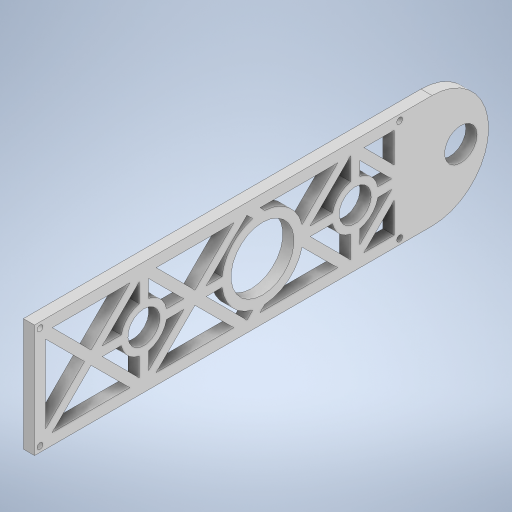
# Autodesk Inventor part: Side_Piece
Saved by Autodesk Inventor 2023 (Build 270158030, 158C)
## iProperties
Created: 2022-06-17
Part Number: Side_Piece
Material: Generic
Document SubType Name: Modeling
Designer: Mlees
Density: 1 g/cm^3
Appearance: Default
Author: Mlees
Autodesk Inventor part; units mm, degrees
ref_plane "YZ Plane" through (0, 0, 0) normal (1, 0, 0) x (0, 1, 0)
ref_plane "XZ Plane" through (0, 0, 0) normal (0, 1, 0) x (-1, 0, 0)
ref_plane "XY Plane" through (0, 0, 0) normal (0, 0, 1) x (1, 0, 0)
sketch "Sketch1" plane through (0, 0, 0) normal (1, 0, 0) x (0, 1, 0)
  line L0 (0, 0) -> (61, 0)
  line L1 (61, 0) -> (61, -200)
  line L2 (61, -200) -> (0, -200)
  line L3 (0, -200) -> (0, 0)
  line L4 (51.4645, -6) -> (9.5355, -6)
  circle A0 centre (30.5, -173) radius 8.625
  circle A1 centre (30.5, -123) radius 17
  circle A2 centre (30.5, -59) radius 8.625
  line L5 (55, -51.4645) -> (55, -9.5355)
  line L6 (55, -9.5355) -> (34.0355, -30.5)
  line L7 (6, -9.5355) -> (26.9645, -30.5)
  line L8 (51.4645, -6) -> (30.5, -26.9645)
  line L9 (26.9645, -30.5) -> (6, -51.4645)
  line L10 (9.5355, -6) -> (30.5, -26.9645)
  line L11 (34.0355, -30.5) -> (55, -51.4645)
  line L12 (6, -9.5355) -> (6, -51.4645)
  line L13 (51.4645, -111.0711) -> (55, -114.6066)
  line L14 (9.5355, -111.0711) -> (6, -114.6066)
  line L15 (55, -107.5355) -> (55, -65.6066)
  line L16 (26.9645, -86.5711) -> (6, -107.5355)
  line L17 (34.0355, -86.5711) -> (55, -107.5355)
  line L18 (55, -65.6066) -> (34.0355, -86.5711)
  line L19 (28, -92.6066) -> (9.5355, -111.0711)
  line L20 (6, -65.6066) -> (26.9645, -86.5711)
  line L21 (33, -92.6066) -> (51.4645, -111.0711)
  line L22 (6, -65.6066) -> (6, -107.5355)
  line L23 (40.9822, -44.5178) -> (52.9645, -56.5)
  line L24 (52.0355, -61.5) -> (33, -80.5355)
  line L25 (28, -80.5355) -> (8.9645, -61.5)
  line L26 (8.0355, -56.5) -> (28, -36.5355)
  line L27 (33, -36.5355) -> (40.9822, -44.5178)
  line L28 (33, -36.5355) -> (33, -46.7526)
  line L29 (33, -71.2474) -> (33, -80.5355)
  line L30 (28, -36.5355) -> (28, -46.7526)
  line L31 (28, -71.2474) -> (28, -80.5355)
  line L32 (18.2526, -61.5) -> (8.9645, -61.5)
  line L33 (18.2526, -56.5) -> (8.0355, -56.5)
  arc A3 (28, -46.7526) -> (18.2526, -56.5) centre (30.5, -59) ccw
  arc A4 (18.2526, -61.5) -> (28, -71.2474) centre (30.5, -59) ccw
  arc A5 (33, -71.2474) -> (42.7474, -61.5) centre (30.5, -59) ccw
  arc A6 (42.7474, -56.5) -> (33, -46.7526) centre (30.5, -59) ccw
  line L34 (52.0355, -61.5) -> (42.7474, -61.5)
  line L35 (52.9645, -56.5) -> (42.7474, -56.5)
  line L36 (10.8223, -175.5) -> (28, -192.6777)
  line L37 (50.1777, -175.5) -> (33, -192.6777)
  line L38 (38.7487, -194) -> (55, -177.7487)
  line L39 (6, -177.7487) -> (22.2513, -194)
  line L40 (9.5355, -167.1421) -> (6.1777, -170.5)
  line L41 (51.4645, -167.1421) -> (54.8223, -170.5)
  line L42 (55, -194) -> (55, -177.7487)
  line L43 (55, -163.6066) -> (55, -121.6777)
  line L44 (6, -194) -> (22.2513, -194)
  line L45 (38.7487, -194) -> (55, -194)
  line L46 (6, -121.6777) -> (6, -163.6066)
  line L47 (6, -177.7487) -> (6, -194)
  line L48 (6, -114.6066) -> (9.1371, -117.7437)
  line L49 (6, -121.6777) -> (8.5334, -124.211)
  line L50 (35.7563, -144.3629) -> (55, -163.6066)
  line L51 (55, -114.6066) -> (51.8629, -117.7437)
  line L52 (25.2437, -144.3629) -> (6, -163.6066)
  line L53 (55, -121.6777) -> (52.4666, -124.211)
  line L54 (28, -148.6777) -> (9.5355, -167.1421)
  line L55 (33, -148.6777) -> (51.4645, -167.1421)
  arc A7 (8.5334, -124.211) -> (25.2437, -144.3629) centre (30.5, -123) ccw
  arc A8 (35.7563, -144.3629) -> (52.4666, -124.211) centre (30.5, -123) ccw
  line L56 (33, -160.7526) -> (33, -148.6777)
  line L57 (33, -185.2474) -> (33, -192.6777)
  line L58 (28, -185.2474) -> (28, -192.6777)
  line L59 (42.7474, -175.5) -> (50.1777, -175.5)
  line L60 (42.7474, -170.5) -> (54.8223, -170.5)
  line L61 (18.2526, -170.5) -> (6.1777, -170.5)
  line L62 (28, -160.7526) -> (28, -148.6777)
  line L63 (18.2526, -175.5) -> (10.8223, -175.5)
  arc A9 (18.2526, -175.5) -> (28, -185.2474) centre (30.5, -173) ccw
  arc A10 (33, -185.2474) -> (42.7474, -175.5) centre (30.5, -173) ccw
  arc A11 (42.7474, -170.5) -> (33, -160.7526) centre (30.5, -173) ccw
  arc A12 (28, -160.7526) -> (18.2526, -170.5) centre (30.5, -173) ccw
  line L64 (33, -92.6066) -> (33, -101.1425)
  line L65 (28, -92.6066) -> (28, -101.1425)
  arc A13 (51.8629, -117.7437) -> (33, -101.1425) centre (30.5, -123) ccw
  arc A14 (28, -101.1425) -> (9.1371, -117.7437) centre (30.5, -123) ccw
  dimension "d0" = 61
  dimension "d1" = 200
  dimension "d49" = 17.25
  dimension "d50" = 34
  dimension "d51" = 17.25
  constraints: 132 end point, 35 parallel, 24 point on circle, 15 centre point, 12 perpendicular, 4 point on line, 3 coincident, 2 vertical, 1 horizontal
  measures "d0" distance of L1.end L2.end
  measures "d1" distance of L0.end L1.end
  measures "d49" diameter of A2
  measures "d50" diameter of A1
  measures "d51" diameter of A0
extrude "Extrusion1" add sketch "Sketch1" along normal blind 6
sketch "Sketch2" plane through (0, 0, 0) normal (-1, 0, 0) x (0, 0, 1)
  line L0 (0, 0) -> (-200, 0) projected
  line L1 (-200, 61) -> (0, 61) projected
  line L2 (-200, 0) -> (-200, 61) projected
  line L3 (0, 61) -> (0, 0) projected
  point P0 (-197, 58)
  point P1 (-197, 3)
  point P2 (-3, 58)
  point P3 (-3, 3)
hole "Hole1" at (0, 58, -3) at (0, 58, -197) at (0, 3, -197) at (0, 3, -3) direction (1, 0, 0) diameter 3.25 depth 6 countersink diameter 5 countersink angle 90
sketch "Sketch3" plane through (6, 0, 0) normal (1, 0, 0) x (0, 0, -1)
  circle A0 centre (173, 30.5) radius 8.625 projected
  circle A1 centre (230, 30.5) radius 2.75
  circle A2 centre (230, 30.5) radius 8.75
  line L0 (200, 0) -> (200, 61) projected
  line L1 (245, 30.5) -> (245, 61)
  line L2 (200, 0) -> (200, 61)
  line L3 (200, 61) -> (245, 61)
  line L4 (245, 30.5) -> (245, 0)
  line L5 (245, 0) -> (200, 0)
  point P0 (0, 0)
  dimension "d53" = 5.5
  dimension "d54" = 17.5
  dimension "d55" = 15
  constraints: 10 end point, 2 centre point, 2 perpendicular, 1 coincident, 1 collinear, 1 vertical
  measures "d53" diameter of A1
  measures "d54" diameter of A2
  measures "d55" distance of A2.centre L1.start
extrude "Extrusion2" add sketch "Sketch3" against normal blind 6 contours L0 L3 L1 L4 L5
fillet "Fillet1" radius 30.5 2 edges at (3, 61, -245) (3, 0, -245)
body "Solid1"
